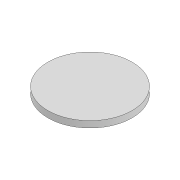
# Autodesk Inventor part: 30_Cube_Z_Focus_MGN_NEMA_timingbelt_v3
Saved by Autodesk Inventor 2022 (Build 260153000, 153)
## iProperties
Created: 2021-12-02
Part Number: 30_Cube_Z_Focus_MGN_NEMA_timingbelt_v3
Material: Generisch
Document SubType Name: Modeling
Designer: diederichbenedict
Density: 1 g/cm^3
Appearance: Vorgabe
Author: diederichbenedict
Autodesk Inventor part; units mm, degrees
ref_plane "YZ Plane" through (0, 0, 0) normal (1, 0, 0) x (0, 1, 0)
ref_plane "XZ Plane" through (0, 0, 0) normal (0, 1, 0) x (-1, 0, 0)
ref_plane "XY Plane" through (0, 0, 0) normal (0, 0, 1) x (1, 0, 0)
sketch "Skizze1" plane through (0, 0, 0) normal (0, 1, 0) x (-1, 0, 0)
  circle A0 centre (0, 0) radius 19.25
  circle A1 centre (0, 0) radius 19.75
  dimension "d0" = 38.5
  dimension "d1" = 0.5
  constraints: 2 centre point, 1 coincident
  measures "d0" diameter of A0
  measures "d1" radial gap between concentric circles of A0 A1
extrude "Extrusion1" add sketch "Skizze1" along normal blind 3
sketch "Skizze2" plane through (0, 3, 0) normal (0, 1, 0) x (1, 0, 0)
  circle A0 centre (0, 0) radius 19.75 projected
  line L0 (-10.9514, -0.5507) -> (-9.9514, -0.5507) construction
  circle A1 centre (0, 0) radius 19.75 projected
  circle A2 centre (0, 0) radius 19.25 projected
  arc A3 (-10.1928, -0.3825) -> (-10.1928, 0.3825) centre (-9.7907, 0) ccw
  circle A4 centre (0, 0) radius 19.25 projected
  arc A5 (-9.9638, 0.85) -> (-9.7216, 0.5507) centre (-9.687, 0.8264) ccw
  arc A6 (-9.7216, -0.5507) -> (-9.9638, -0.85) centre (-9.687, -0.8264) ccw
  point P0 (-9.9865, 0.5193)
  point P1 (-9.9865, -0.5193)
  point P2 (-9.9865, 0.5193)
  point P3 (-9.9865, -0.5193)
  point P4 (-9.9638, 0.85)
  dimension "d9" = 1.11
  dimension "d10" = 0
  dimension "d11" = 1.7
  dimension "d12" = 0.85
  dimension "d14" = 9.7907
  constraints: 10 point on circle, 3 centre point, 2 coincident, 2 end point, 2 tangent, 1 horizontal, 1 point on line, 11 other
  measures "d9" diameter of A3
  measures "d10" vertical distance of point (0, 0) A3.centre
  measures "d11" distance of A6.end A5.start
  measures "d12" vertical distance of A5.start A3.centre
  measures "d14" distance of point (0, 0) A3.centre
extrude "Extrusion2" add sketch "Skizze2" against normal up to surface (3 mm away) contours A2
pattern_circular "Runde Anordnung1" count 31 over 360 about axis through (0, 0, 0) along (0, 1, 0) of "Extrusion2"
equation "\"d12\" = 0.5 * d11"
